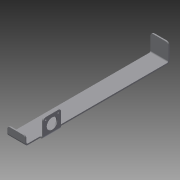
# Autodesk Inventor part: Arm
Saved by Autodesk Inventor 2015 (Build 190159000, 159)
## iProperties
Created: 2015-12-09
Part Number: Arm
Material: Generic
Document SubType Name: Sheet Metal
Designer: Nick
Density: 1 g/cm^3
Sheet Metal Rule: Default
Appearance: Default
Author: Nick
Autodesk Inventor part; units mm, degrees
ref_plane "YZ Plane" through (0, 0, 0) normal (1, 0, 0) x (0, 1, 0)
ref_plane "XZ Plane" through (0, 0, 0) normal (0, 1, 0) x (-1, 0, 0)
ref_plane "XY Plane" through (0, 0, 0) normal (0, 0, 1) x (1, 0, 0)
sketch "Sketch1" plane through (0, 0, 0) normal (0, 1, 0) x (-1, 0, 0)
  line L0 (0, 0) -> (0, -327.3552)
  line L1 (0, -327.3552) -> (42.291, -327.3552)
  line L2 (42.291, -327.3552) -> (42.291, 0)
  line L3 (42.291, 0) -> (0, 0)
  line L4 (42.291, -327.3552) -> (42.291, -336.7024)
  line L5 (42.291, -336.7024) -> (0, -336.7024)
  line L6 (0, -336.7024) -> (0, -327.3552)
  line L7 (42.291, 0) -> (42.291, 9.3472)
  line L8 (42.291, 9.3472) -> (0, 9.3472)
  line L9 (0, 9.3472) -> (0, 0)
  line L10 (0, 0) -> (0, -27.9146)
  line L11 (0, -27.9146) -> (-9.3472, -27.9146)
  line L12 (-9.3472, -27.9146) -> (-9.3472, -70.2056)
  line L13 (-9.3472, -70.2056) -> (0, -70.2056)
  line L14 (-9.3472, -27.9146) -> (-39.0144, -27.9146)
  line L15 (-39.0144, -27.9146) -> (-39.0144, -70.2056)
  line L16 (-39.0144, -70.2056) -> (-9.3472, -70.2056)
  line L17 (-39.0144, -27.9146) -> (-39.0144, -27.9146)
  line L18 (-45.3644, -34.2646) -> (-45.3644, -63.8556)
  line L19 (-39.0144, -70.2056) -> (-39.0144, -70.2056)
  arc A0 (-39.0144, -27.9146) -> (-45.3644, -34.2646) centre (-39.0144, -34.2646) ccw
  arc A1 (-45.3644, -63.8556) -> (-39.0144, -70.2056) centre (-39.0144, -63.8556) ccw
  line L20 (0, 9.3472) -> (0, 17.0434)
  line L21 (0, 17.0434) -> (42.291, 17.0434)
  line L22 (42.291, 17.0434) -> (42.291, 9.3472)
  line L23 (42.291, 17.0434) -> (42.291, 17.0434)
  line L24 (35.941, 23.3934) -> (6.35, 23.3934)
  line L25 (0, 17.0434) -> (0, 17.0434)
  arc A2 (6.35, 23.3934) -> (0, 17.0434) centre (6.35, 17.0434) ccw
  arc A3 (42.291, 17.0434) -> (35.941, 23.3934) centre (35.941, 17.0434) ccw
  line L26 (0, -336.7024) -> (0, -366.3696)
  line L27 (0, -366.3696) -> (42.291, -366.3696)
  line L28 (42.291, -366.3696) -> (42.291, -336.7024)
  line L29 (42.291, -366.3696) -> (42.291, -366.3696)
  line L30 (35.941, -372.7196) -> (6.35, -372.7196)
  line L31 (0, -366.3696) -> (0, -366.3696)
  arc A4 (35.941, -372.7196) -> (42.291, -366.3696) centre (35.941, -366.3696) ccw
  arc A5 (0, -366.3696) -> (6.35, -372.7196) centre (6.35, -366.3696) ccw
  circle A6 centre (-39.0144, -34.2646) radius 1.4859
  circle A7 centre (-39.0144, -63.8556) radius 1.4859
  circle A8 centre (-24.5364, -49.0601) radius 12.7
  line L32 (-4.6736, -27.9146) -> (-4.6736, -70.2056)
  line L33 (42.291, 4.6736) -> (0, 4.6736)
  line L34 (42.291, -332.0288) -> (0, -332.0288)
  point P0 (-45.3644, -27.9146)
  point P1 (-45.3644, -70.2056)
  point P2 (42.291, 23.3934)
  point P3 (42.291, -372.7196)
  point P4 (0, -372.7196)
  point P5 (-45.3644, -49.0601)
  dimension "d0" = 327.3552
  dimension "d1" = 42.291
  dimension "d2" = 9.3472
  dimension "d3" = 9.3472
  dimension "d4" = 27.9146
  dimension "d5" = 9.3472
  dimension "d6" = 42.291
  dimension "d7" = 29.6672
  dimension "d8" = 6.35
  dimension "d9" = 6.35
  dimension "d10" = 7.6962
  dimension "d11" = 6.35
  dimension "d12" = 6.35
  dimension "d13" = 29.6672
  dimension "d14" = 6.35
  dimension "d15" = 6.35
  dimension "d16" = 2.9718
  dimension "d17" = 2.9718
  dimension "d18" = 25.4
  dimension "d19" = 0
  dimension "d20" = 20.828
  constraints: 70 end point, 20 perpendicular, 19 point on line, 12 point on circle, 12 tangent, 9 centre point, 7 midpoint, 5 vertical, 3 equal radius, 2 coincident, 2 parallel, 1 horizontal
  measures "d0" distance of L0.start L0.end
  measures "d1" distance of L0.end L1.end
  measures "d2" distance of L1.end L4.end
  measures "d3" distance of L2.end L7.end
  measures "d4" distance of L0.start L10.end
  measures "d5" distance of L10.end L11.end
  measures "d6" distance of L11.end L12.end
  measures "d7" distance of L11.end L14.end
  measures "d8" distance of L14.end point (-45.364, -27.915)
  measures "d9" radius of A0
  measures "d10" distance of L8.end L20.end
  measures "d11" distance of L21.end point (42.291, 23.393)
  measures "d12" radius of A2
  measures "d13" distance of L5.end L26.end
  measures "d14" distance of L27.end point (42.291, -372.72)
  measures "d15" radius of A4
  measures "d16" diameter of A6
  measures "d17" diameter of A7
  measures "d18" diameter of A8
  measures "d19" vertical distance of point (-45.364, -49.06) A8.centre
  measures "d20" distance from line of L18 A8.centre
extrude "Plate1" add sketch "Sketch1" along normal blind 3.048
extrude "Cut1" cut sketch "Sketch1" along normal blind 3.048 contours A6 L15 | L15 A6 | A7 L15 | L15 A7
fold "Fold1" angle 90 bend radius 3.048 thickness 3.048 k factor 0.44 line from (4.6736, 0, -27.9146) to (4.6736, 0, -70.2056) line at bend centre moving side (1, 0, 0) folds toward (0, 1, 0)
fold "Fold2" angle 90 bend radius 3.048 thickness 3.048 k factor 0.44 line from (-42.291, 0, -332.0288) to (0, 0, -332.0288) line at bend centre moving side (0, 0, -1) folds toward (0, 1, 0)
fold "Fold3" angle 90 bend radius 3.048 thickness 3.048 k factor 0.44 line from (-42.291, 0, 4.6736) to (0, 0, 4.6736) line at bend centre moving side (0, 0, 1) folds toward (0, 1, 0)
equation "\"d22\" = Thickness"
equation "\"d24\" = BendReliefWidth"
equation "\"d25\" = BendReliefDepth"
equation "\"d26\" = MinimumRemnant"
equation "\"d27\" = BendRadius"
equation "\"d29\" = BendRadius"
equation "\"d30\" = BendReliefWidth"
equation "\"d31\" = BendReliefDepth"
equation "\"d32\" = MinimumRemnant"
equation "\"d33\" = BendRadius"
equation "\"d35\" = BendRadius"
equation "\"d36\" = BendReliefWidth"
equation "\"d37\" = BendReliefDepth"
equation "\"d38\" = MinimumRemnant"
equation "\"d39\" = BendRadius"
equation "\"d41\" = BendRadius"
equation "\"BendRadius\" = Thickness"
equation "\"BendReliefWidth\" = Thickness"
equation "\"BendReliefDepth\" = 0.5 * Thickness"
equation "\"CornerReliefSize\" = 4 * Thickness"
equation "\"MinimumRemnant\" = 2 * Thickness"
equation "\"TransitionRadius\" = BendRadius"
equation "\"JacobiRadiusSize\" = BendRadius"
equation "\"GapSize\" = Thickness"
equation "\"d21\" = BendRadius"
equation "\"Thickness\" = 3.048"
body "Solid1"
